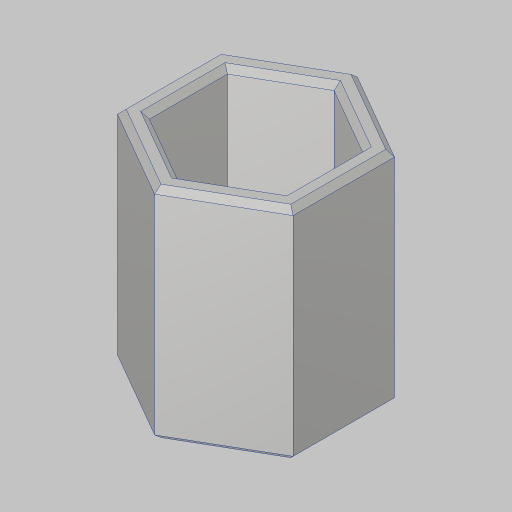
# Autodesk Inventor part: 0_5_Hex_0_375_Hex_Adapter
Saved by Autodesk Inventor 2023.5 (Build 275446000, 446)
## iProperties
Created: 2025-02-23
Part Number: 0_5_Hex_0_375_Hex_Adapter
Material: Aluminum 6061
Document SubType Name: Modeling
Designer: slick
Density: 2.7 g/cm^3
Appearance: Aluminum - Flat
Author: slick
Autodesk Inventor part; units mm, degrees
ref_plane "YZ Plane" through (0, 0, 0) normal (1, 0, 0) x (0, 1, 0)
ref_plane "XZ Plane" through (0, 0, 0) normal (0, 1, 0) x (-1, 0, 0)
ref_plane "XY Plane" through (0, 0, 0) normal (0, 0, 1) x (1, 0, 0)
sketch "Sketch1" plane through (0, 0, 0) normal (0, 1, 0) x (-1, 0, 0)
  line L0 (6.35, -3.6662) -> (0, -7.3323)
  line L1 (0, -7.3323) -> (-6.35, -3.6662)
  line L2 (-6.35, -3.6662) -> (-6.35, 3.6662)
  line L3 (-6.35, 3.6662) -> (0, 7.3323)
  line L4 (0, 7.3323) -> (6.35, 3.6662)
  line L5 (6.35, 3.6662) -> (6.35, -3.6662)
  line L6 (-4.8895, 2.823) -> (0, 5.6459)
  line L7 (0, 5.6459) -> (4.8895, 2.823)
  line L8 (4.8895, 2.823) -> (4.8895, -2.823)
  line L9 (4.8895, -2.823) -> (0, -5.6459)
  line L10 (0, -5.6459) -> (-4.8895, -2.823)
  line L11 (-4.8895, -2.823) -> (-4.8895, 2.823)
  point P0 (0, 0)
  point P1 (0, 0)
  point P2 (0, 0)
  dimension "d0" = 9.779
  dimension "d1" = 12.7
  constraints: 24 end point, 2 coincident, 2 vertical, 26 other
  measures "d0" distance between parallel lines of L8 L11
  measures "d1" distance between parallel lines of L2 L5
extrude "Extrusion1" add sketch "Sketch1" along normal blind 15.875
chamfer "Chamfer1" distance 0.4 angle 45 24 edges at (-3.175, 0, 5.4993) (3.175, 0, 5.4993) (6.35, 0, 0) (3.175, 0, -5.4993) (-3.175, 0, -5.4993) (-6.35, 0, 0) (-2.4447, 0, -4.2344) (2.4448, 0, -4.2344) (4.8895, 0, 0) (2.4447, 0, 4.2344) (-2.4447, 0, 4.2344) (-4.8895, 0, 0) (-4.8895, 15.875, 0) (-2.4447, 15.875, 4.2344) (2.4447, 15.875, 4.2344) (4.8895, 15.875, 0) (2.4448, 15.875, -4.2344) (-2.4447, 15.875, -4.2344) (-3.175, 15.875, -5.4993) (-6.35, 15.875, 0) (-3.175, 15.875, 5.4993) (3.175, 15.875, 5.4993) (6.35, 15.875, 0) (3.175, 15.875, -5.4993)
body "Solid1"
